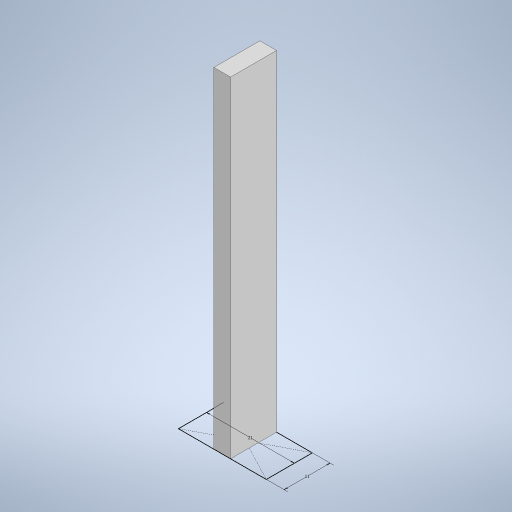
# Autodesk Inventor part: 부품1
Saved by Autodesk Inventor 2024 (Build 280153000, 153)
## iProperties
Created: 2024-07-10
Part Number: 부품1
Material: 일반
Document SubType Name: Modeling
Designer: Gihyeok Na
Density: 1 g/cm^3
Appearance: 기본값
Author: Gihyeok Na
Autodesk Inventor part; units mm, degrees
ref_plane "YZ Plane" through (0, 0, 0) normal (1, 0, 0) x (0, 1, 0)
ref_plane "XZ Plane" through (0, 0, 0) normal (0, 1, 0) x (-1, 0, 0)
ref_plane "XY Plane" through (0, 0, 0) normal (0, 0, 1) x (1, 0, 0)
sketch "스케치4" plane through (0, 0, 0) normal (0, 1, 0) x (-1, 0, 0)
  line L0 (-2, 5.5) -> (-2, -5.5)
  line L1 (-2, -5.5) -> (2, -5.5)
  line L2 (2, -5.5) -> (2, 5.5)
  line L3 (2, 5.5) -> (-2, 5.5)
  line L4 (-2, 5.5) -> (2, -5.5) construction
  line L5 (-2, -5.5) -> (2, 5.5) construction
  point P0 (0, 0)
  dimension "d12" = 11
  dimension "d13" = 4
  constraints: 12 end point, 2 midpoint, 2 parallel, 1 perpendicular, 1 vertical
  measures "d12" distance of L0.start L0.end
  measures "d13" distance of L1.end L0.end
extrude "돌출3" add sketch "스케치4" along normal blind 79
sketch "스케치5" plane through (0, 0, 0) normal (0, -1, 0) x (1, 0, 0)
  line L0 (-10.5, -5.5) -> (10.5, -5.5)
  line L1 (10.5, -5.5) -> (10.5, 5.5)
  line L2 (10.5, 5.5) -> (-10.5, 5.5)
  line L3 (-10.5, 5.5) -> (-10.5, -5.5)
  line L4 (-10.5, -5.5) -> (10.5, 5.5) construction
  line L5 (10.5, -5.5) -> (-10.5, 5.5) construction
  point P0 (0, 0)
  dimension "d16" = 21
  dimension "d17" = 11
  constraints: 12 end point, 2 midpoint, 2 parallel, 1 horizontal, 1 perpendicular
  measures "d16" distance of L0.start L0.end
  measures "d17" distance of L1.end L0.end
